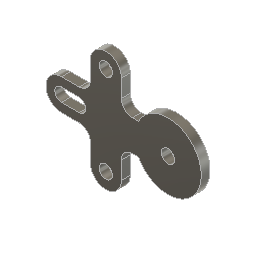
SteeringRodServoAttachment (Autodesk Fusion 360 design; units mm, degrees)
Autodesk Fusion 360 part; units mm, degrees
note: some values were not read from the file. Set by a fixed rule: which sketch regions a step uses.
sketch "Sketch1" plane through (0, 0, 0) normal (0, 0, 1) x (1, 0, 0)
  line L0 (3, 6) -> (38, 6)
  line L1 (38, 6) -> (38, -1)
  line L2 (38, -1) -> (3, -1)
  line L3 (3, -1) -> (3, 6)
  line L4 (3, 6) -> (5, 6)
  line L5 (5, 6) -> (5, -1)
  line L6 (5, -1) -> (3, -1)
  line L7 (3, -1) -> (3, 6)
  line L8 (5, 2.5) -> (12, 2.5)
  line L9 (12, 2.5) -> (12, 4)
  line L10 (12, 4) -> (5, 4)
  line L11 (5, 4) -> (5, 2.5)
  line L12 (5, 2.5) -> (12, 2.5)
  line L13 (12, 2.5) -> (12, 1)
  line L14 (12, 1) -> (5, 1)
  line L15 (5, 1) -> (5, 2.5)
  circle A0 centre (6.5, 2.5) radius 1.5
  circle A1 centre (10.5, 2.5) radius 1.5
  line L16 (3, -1) -> (13, -1)
  line L17 (13, -1) -> (13, 6)
  line L18 (13, 6) -> (3, 6)
  line L19 (3, 6) -> (3, -1)
  line L20 (13, 2.5) -> (20, 2.5)
  line L21 (20, 2.5) -> (20, 16)
  line L22 (20, 16) -> (13, 16)
  line L23 (13, 16) -> (13, 2.5)
  line L24 (13, 2.5) -> (20, 2.5)
  line L25 (20, 2.5) -> (20, -11)
  line L26 (20, -11) -> (13, -11)
  line L27 (13, -11) -> (13, 2.5)
  line L28 (20, 16) -> (20, 14)
  line L29 (13, 14) -> (13, 16)
  line L30 (13, -11) -> (20, -11)
  line L31 (20, -11) -> (20, -9)
  line L32 (13, -9) -> (13, -11)
  line L33 (20, -11) -> (20, -4)
  line L34 (20, -4) -> (13, -4)
  line L35 (13, -4) -> (13, -11)
  circle A2 centre (16.5, -7.5) radius 3.5
  circle A3 centre (16.5, -7.5) radius 1.5
  line L36 (13, 16) -> (20, 16)
  line L37 (20, 16) -> (20, 9)
  line L38 (20, 9) -> (13, 9)
  line L39 (13, 9) -> (13, 16)
  circle A4 centre (16.5, 12.5) radius 3.5
  circle A5 centre (16.5, 12.5) radius 1.5
  line L40 (38, 2.5) -> (23, 2.5)
  line L41 (23, 2.5) -> (23, 10)
  line L42 (23, 10) -> (38, 10)
  line L43 (38, 10) -> (38, 2.5)
  line L44 (23, 2.5) -> (38, 2.5)
  line L45 (38, 2.5) -> (38, -5)
  line L46 (38, -5) -> (23, -5)
  line L47 (23, -5) -> (23, 2.5)
  circle A6 centre (30.5, 2.5) radius 7.5
  circle A7 centre (30.5, 2.5) radius 1.5
  circle A8 centre (22.5, -3.5) radius 2.5
  circle A9 centre (22.5, 8.5) radius 2.5
  circle A10 centre (6.5, 2.5) radius 3.5
  circle A11 centre (10.5, 8.5) radius 2.5
  circle A12 centre (10.5, -3.5) radius 2.5
  dimension "d1" = 35
  dimension "d2" = 7
  dimension "d3" = 2
  dimension "d4" = 7
  dimension "d5" = 1.5
  dimension "d6" = 3
  dimension "d7" = 3
  dimension "d10" = 10
  dimension "d11" = 7
  dimension "d12" = 13.5
  dimension "d13" = 13.5
  dimension "d17" = 7
  dimension "d18" = 3
  dimension "d19" = 7
  dimension "d20" = 3
  dimension "d21" = 15
  dimension "d22" = 7.5
  dimension "d23" = 7.5
  dimension "d24" = 15
  dimension "d25" = 3
  dimension "d26" = 5
  dimension "d27" = 5
  dimension "d30" = 7
  dimension "d31" = 5
  dimension "d32" = 5
  constraint horizontal L0
  constraint vertical L1
  constraint horizontal L2
  constraint vertical L3
  constraint horizontal L4
  constraint vertical L5
  constraint horizontal L6
  constraint vertical L7
  constraint horizontal L8
  constraint vertical L9
  constraint horizontal L10
  constraint vertical L11
  constraint midpoint L5 L8.start
  constraint horizontal L12
  constraint vertical L13
  constraint horizontal L14
  constraint vertical L15
  constraint coincident L8.start A0
  constraint coincident L8.end A1
  constraint horizontal L16
  constraint vertical L17
  constraint horizontal L18
  constraint vertical L19
  constraint horizontal L20
  constraint vertical L21
  constraint vertical L23
  constraint midpoint L17 L20.start
  constraint horizontal L24
  constraint vertical L25
  constraint horizontal L26
  constraint vertical L27
  constraint coincident L21 L28.end
  constraint horizontal L30
  constraint vertical L31
  constraint vertical L32
  constraint coincident L25 L31.end
  constraint vertical L33
  constraint horizontal L34
  constraint vertical L35
  constraint coincident L25 L33.end
  constraint tangent L35 A2
  constraint concentric A2 A3
  constraint horizontal L36
  constraint vertical L37
  constraint horizontal L38
  constraint vertical L39
  constraint tangent L37 A4
  constraint concentric A4 A5
  constraint horizontal L40
  constraint vertical L41
  constraint horizontal L42
  constraint vertical L43
  constraint midpoint L1 L40.start
  constraint horizontal L44
  constraint vertical L45
  constraint horizontal L46
  constraint vertical L47
  constraint midpoint L44 A6.centre
  constraint concentric A6 A7
  constraint tangent A6 A8
  constraint tangent L25 A8
  constraint tangent A6 A9
  constraint tangent L21 A9
  constraint concentric A0 A10
  constraint tangent L23 A11
  constraint tangent L18 A11
  constraint tangent L16 A12
  constraint tangent L27 A12
  measures "d1" distance of L0.start L0.end
  measures "d2" distance of L0.start L2.end
  measures "d3" distance of L0.start L4.end
  measures "d4" distance of L8.start L8.end
  measures "d5" distance of L8.start L10.end
  measures "d6" diameter of A0
  measures "d7" diameter of A1
  measures "d10" distance of L2.end L16.end
  measures "d11" distance of L20.start L20.end
  measures "d12" distance of L20.start L22.end
  measures "d13" distance of L20.start L26.end
  measures "d17" distance of L26.end L34.end
  measures "d18" diameter of A3
  measures "d19" distance of L22.end L38.end
  measures "d20" diameter of A5
  measures "d21" distance of L40.start L40.end
  measures "d22" distance of L40.start L42.end
  measures "d23" distance of L40.end L46.end
  measures "d24" diameter of A6
  measures "d25" diameter of A7
  measures "d26" diameter of A8
  measures "d27" diameter of A9
  measures "d30" diameter of A10
  measures "d31" diameter of A11
  measures "d32" diameter of A12
extrude "Extrude1" add sketch "Sketch1" along normal blind 2 contours L0 L3 L4 L5 L7 L18 L19 A10 | L0 L5 L18 A10 | L2 L3 L5 L6 L7 L16 L19 A10 | L5 L11 L15 A10 | L0 L2 L9 L10 L13 L14 L16 L17 L18 L23 L27 A10 | L5 L10 A10 | L2 L5 L16 A10 | L5 L14 A10 | L5 L10 L11 A0 | L5 L14 L15 A0 | L0 L21 L23 L38 | L0 L17 L20 L21 L23 L24 | L9 L10 A1 | L0 L21 A9 | L0 L2 L21 L25 L41 L47 | L2 L17 L20 L24 L25 L27 | L23 L38 L39 A4 | L13 L14 A1 | L2 L25 L27 L34 | A4 | L21 L37 L38 A4 | L2 L25 A8 | L27 L34 L35 A2 | L0 L41 A6 | A2 | L25 L33 L34 A2 | L0 A6 | L0 L40 L44 A6 A7 | L2 L47 A6 | L2 L40 L44 A6 A7 | L2 A6
extrude "Extrude2" add sketch "Sketch1" along normal blind 2 contours L2 L16 L27 A12
extrude "Extrude3" add sketch "Sketch1" along normal blind 2 contours L0 L18 L23 A11
extrude "Extrude4" cut sketch "Sketch1" along normal blind 2 contours L0 L3 L4 L5 L7 L18 L19 A10
extrude "Extrude5" cut sketch "Sketch1" along normal blind 2 contours L0 L5 L18 A10 | L2 L3 L5 L6 L7 L16 L19 A10 | L2 L5 L16 A10
